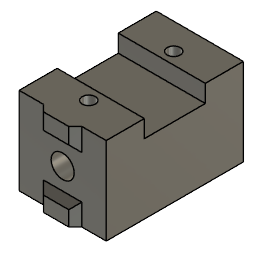
Gantry Limit Switch Bracket (Autodesk Fusion 360 design; units mm, degrees)
part number: 2026-06-20-08-30-52-677
Autodesk Fusion 360 part; units mm, degrees
sketch "Sketch1" plane through (0, 0, 0) normal (0, 0, 1) x (1, 0, 0)
  line L0 (10, -7) -> (-10, -7)
  line L1 (-10, 7) -> (10, 7)
  line L2 (5, 7) -> (-5, -7) construction
  line L3 (5, -7) -> (-5, 7) construction
  line L4 (10, 0) -> (-10, 0) construction
  line L5 (0, -9.75) -> (0, 9.75) construction
  circle A0 centre (0, -9.75) radius 1.5
  circle A1 centre (0, 9.75) radius 1.5
  line L6 (-10, -15.75) -> (10, -15.75)
  line L7 (-10, 15.75) -> (10, 15.75)
  line L8 (-10, -15.75) -> (-10, 15.75)
  line L9 (10, -15.75) -> (10, 15.75)
  dimension "d1" = 14
  dimension "d2" = 10
  dimension "d3" = 3
  dimension "d4" = 3
  dimension "d5" = 19.5
  dimension "d6" = 20
  constraint parallel L0 L1
  constraint coincident L2 origin
  constraint coincident L3 origin
  constraint perpendicular L1 L5
  constraint midpoint origin L5
  constraint coincident L5.start A0.centre
  constraint coincident L5.end A1.centre
  constraint midpoint origin L4
  constraint perpendicular L5 L6
  constraint perpendicular L4 L8
  constraint coincident L4.start L9
  constraint coincident L4.end L8
  constraint coincident L8 L1.start
  constraint coincident L3.end L1
  constraint coincident L8 L0.end
  constraint coincident L2.end L0
  constraint coincident L9 L0.start
  constraint coincident L3.start L0
  constraint coincident L9 L1.end
  constraint coincident L2.start L1
  measures "d1" distance of L2.end L3.end
  measures "d2" distance of L3.start L2.end
  measures "d3" diameter of A0
  measures "d4" diameter of A1
  measures "d5" distance of L5.start L5.end
  measures "d6" distance of L4.start L4.end
extrude "Extrude1" add sketch "Sketch1" along normal blind 20 contours L0 L6 L8 L9 | L1 L7 L8 L9 makes body 1 at (-3.3333, -15.75, 6.6667) makes body 2 at (-3.3333, 7, 6.6667)
extrude "Extrude2" add sketch "Sketch1" along normal blind 16 contours L0 L1 L8 L9 bodies 1 2
sketch "Sketch2" plane through (0, -15.75, 0) normal (0, -1, 0) x (1, 0, 0)
  line L0 (-10, 0) -> (10, 0)
  line L1 (10, 0) -> (10, 20)
  line L2 (10, 20) -> (-10, 20)
  line L3 (-10, 20) -> (-10, 0)
  circle A0 centre (0, 9.8899) radius 2.65
  dimension "d11" = 5.3
  measures "d11" diameter of A0
extrude "Extrude3" add sketch "Sketch1" along normal blind 14 contours A0 | A1 bodies 1
extrude "Extrude4" cut sketch "Sketch2" against normal blind 31.5 contours A0 bodies 1
sketch "Sketch3" plane through (0, 0, 0) normal (0, 0, 1) x (1, 0, 0)
  line L0 (-10, -15.75) -> (-10, 15.75)
  line L1 (10, -15.75) -> (10, 15.75)
  line L2 (-2.9, -17.25) -> (2.9, -17.25)
  line L3 (2.9, -15.75) -> (2.9, -17.25)
  line L4 (-2.9, -15.75) -> (-2.9, -17.25)
  line L5 (-10, -15.75) -> (-2.9, -15.75)
  line L6 (2.9, -15.75) -> (10, -15.75)
  line L7 (-2.9, -15.75) -> (2.9, -15.75)
  line L8 (-10, -15.75) -> (10, -15.75)
  line L9 (0, 0) -> (0, -34.5) construction
  dimension "d23" = 1.5
  dimension "d27" = 5.8
  constraint collinear L5 L6
  constraint perpendicular L3 L7
  constraint coincident L9.start origin
  constraint perpendicular L2 L9
  constraint midpoint L2 L9
  measures "d23" distance of L2 L8
  measures "d27" distance of L3 L4
extrude "Extrude5" add sketch "Sketch3" along normal blind 20 bodies 1
extrude "Extrude6" cut sketch "Sketch2" along normal blind 3 contours A0 bodies 1
chamfer "Chamfer1" distance 1.5 angle 45 1 edges at (2.9, -15.75, 10) on bodies 1
chamfer "Chamfer1" distance 1.5 angle 45 1 edges at (-2.9, -15.75, 10) on bodies 1
sketch "Sketch4" plane through (0, 15.75, 0) normal (0, 1, 0) x (-1, 0, 0)
  circle A0 centre (0, 9.8899) radius 2.65
  line L0 (-10, 0) -> (10, 0)
  line L1 (10, 0) -> (10, 20)
  line L2 (10, 20) -> (-10, 20)
  line L3 (-10, 20) -> (-10, 0)
  circle A1 centre (0, 9.8899) radius 5
  dimension "d24" = 10
  constraint concentric A0 A1
  measures "d24" diameter of A1
extrude "Extrude7" cut sketch "Sketch4" against normal blind 5 contours A1 bodies 1
sketch "Sketch5" plane through (0, 0, 0) normal (0, 0, 1) x (1, 0, 0)
  line L0 (2.65, -17.25) -> (-2.65, -17.25)
  line L1 (2.65, -17.25) -> (-2.65, -17.25)
sketch "Sketch6" plane through (0, -15.75, 0) normal (0, -1, 0) x (1, 0, 0)
  line L0 (4.7787, 4.9544) -> (-4.7787, 4.9544)
  line L1 (-4.7787, 4.9544) -> (-4.7787, 16.3254)
  line L2 (-4.7787, 16.3254) -> (4.7787, 16.3254)
  line L3 (4.7787, 16.3254) -> (4.7787, 4.9544)
  point P0 (0, 9.8899)
  point P1 (0, 9.8899)
  constraint horizontal L0
  constraint perpendicular L0 L1
  constraint parallel L0 L2
  constraint parallel L1 L3
  constraint coincident P0 P1
extrude "Extrude8" cut sketch "Sketch6" along normal blind 1.5 bodies 1
chamfer "Chamfer2" distance 1.5 angle 45 1 edges at (0, -15.75, 16.3254) on bodies 1
chamfer "Chamfer3" distance 1.5 angle 45 1 edges at (0, -17.25, 4.9544) on bodies 1
named bodies: "Gantry Limit Switch Bracket"
